DHECbottomlockouterringv2 (Autodesk Fusion 360 design; units mm, degrees)
Autodesk Fusion 360 part; units mm, degrees
note: some values were not read from the file. Chosen so that the rebuilt part matches the saved one: a direction.
sketch "Sketch1" plane through (0, 0, 0) normal (1, 0, 0) x (0, 1, 0)
  line L0 (44.3, 0) -> (47.3, 0)
  line L1 (47.3, 0) -> (47.3, 15)
  line L2 (47.3, 15) -> (37.8, 15)
  line L3 (37.8, 15) -> (37.8, 10)
  line L4 (37.8, 10) -> (44.3, 10)
  line L5 (44.3, 10) -> (44.3, 0)
  dimension "d1" = 3
  dimension "d2" = 6.5
  dimension "d3" = 44.3
  dimension "d4" = 10
  dimension "d5" = 5
  constraint horizontal L0
  constraint perpendicular L0 L1
  constraint perpendicular L1 L2
  constraint perpendicular L2 L3
  constraint perpendicular L3 L4
  constraint perpendicular L0 L5
  constraint coincident origin L0
  measures "d1" distance of L1 L5
  measures "d2" distance of L3.end L4.end
  measures "d3" distance of origin L5
  measures "d4" distance of L0 L4
  measures "d5" distance of L2 L4
revolve "Revolve1" add sketch "Sketch1" angle 360 about axis through (0, 0, 1.75) along (0, 0, 1)
sketch "Sketch2" plane through (0, 0, 15) normal (0, 0, 1) x (-1, 0, 0)
  circle A0 centre (0, 0) radius 37.8
  circle A1 centre (0, 0) radius 47.3
  line L0 (46.2308, -10) -> (38.7308, -10)
  line L1 (38.7308, -10) -> (38.7308, 10)
  line L2 (38.7308, 10) -> (46.2308, 10)
  line L3 (46.2308, 10) -> (46.2308, -10)
  line L4 (-38.7308, -10) -> (-46.2308, -10)
  line L5 (-46.2308, -10) -> (-46.2308, 10)
  line L6 (-46.2308, 10) -> (-38.7308, 10)
  line L7 (-38.7308, 10) -> (-38.7308, -10)
  dimension "d7" = 7.5
  dimension "d8" = 20
  constraint horizontal L0
  constraint vertical L1
  constraint horizontal L2
  constraint vertical L3
  constraint coincident A1 L0.start
  constraint horizontal L4
  constraint vertical L5
  constraint horizontal L6
  constraint vertical L7
  constraint equal L0 L4
  constraint equal L1 L7
  constraint coincident A1 L4.end
  constraint coincident A1 L5.end
  constraint coincident A1 L2.end
  measures "d7" distance of L5.end L6.end
  measures "d8" distance of L4 L6
extrude "Extrude1" add sketch "Sketch2" along normal blind 20 contours L0 L1 L2 L3 | L4 L5 L6 L7
sketch "Sketch3" plane through (46.2308, 0, 0) normal (1, 0, 0) x (0, 1, 0)
  line L0 (-10, 15) -> (10, 15)
  line L1 (10, 15) -> (10, 35)
  line L2 (10, 35) -> (-10, 35)
  line L3 (-10, 35) -> (-10, 15)
  circle A0 centre (0, 25) radius 10
  circle A1 centre (0, 25) radius 3.5
  dimension "d11" = 7
  constraint tangent L2 A0
  constraint concentric A0 A1
  constraint tangent L3 A0
  constraint tangent L1 A0
  measures "d11" diameter of A1
extrude "Extrude2" cut sketch "Sketch3" against normal through all contours L2 L3 A0 | L1 L2 A0 | A1
